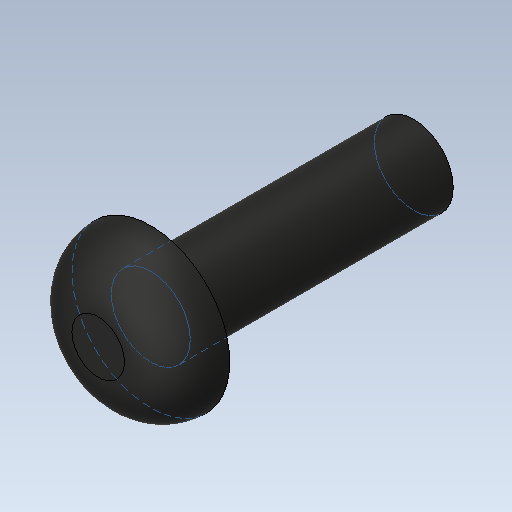
# Autodesk Inventor part: M3ボタンボルト10
Saved by Autodesk Inventor 2020 (Build 240168000, 168)
## iProperties
Created: 2016-02-25
Part Number: M3ボタンボルト10
Material: 鋼、高強度、低合金
Document SubType Name: Modeling
Designer: Riku
Density: 7.85 g/cm^3
Appearance: 鉄黒
Mass: 0.890688 g
Surface Area: 1.70536 cm^2
Volume: 0.113463 cm^3
Author: Riku
Autodesk Inventor part; units mm, degrees
ref_plane "YZ Plane" through (0, 0, 0) normal (1, 0, 0) x (0, 1, 0)
ref_plane "XZ Plane" through (0, 0, 0) normal (0, 1, 0) x (-1, 0, 0)
ref_plane "XY Plane" through (0, 0, 0) normal (0, 0, 1) x (1, 0, 0)
sketch "スケッチ1" plane through (0, 0, 0) normal (0, 0, 1) x (1, 0, 0)
  circle A0 centre (0, 0) radius 1.5
  dimension "d0" = 3
  constraints: 1 centre point, 1 coincident
  measures "d0" diameter of A0
extrude "押し出し1" add sketch "スケッチ1" along normal blind 10
sketch "スケッチ2" plane through (0, 0, 10) normal (0, 0, 1) x (1, 0, 0)
  circle A0 centre (0, 0) radius 1.5 projected
  circle A1 centre (0, 0) radius 3
  dimension "d3" = 6
  constraints: 1 centre point, 1 coincident
  measures "d3" diameter of A1
extrude "押し出し2" add sketch "スケッチ2" along normal blind 2 contours A0 | A1
fillet "フィレット1" radius 2 1 edges at (-3, 0, 12)
